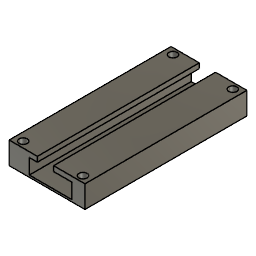
Rail (Autodesk Fusion 360 design; units mm, degrees)
part number: 2025-11-19-14-05-20-306
Autodesk Fusion 360 part; units mm, degrees
sketch "Sketch1" plane through (0, 0, 0) normal (0, 0, 1) x (1, 0, 0)
  line L0 (0, 0) -> (95.25, 0)
  line L1 (95.25, 0) -> (95.25, 203.2)
  line L2 (95.25, 203.2) -> (0, 203.2)
  line L3 (0, 203.2) -> (0, 0)
  dimension "d1" = 95.25
  dimension "d2" = 203.2
  constraint horizontal L0
  constraint vertical L1
  constraint horizontal L2
  constraint vertical L3
  constraint coincident L0.start L3.end
  measures "d1" distance of L0.start L0.end
  measures "d2" distance of L0.start L2.end
extrude "Extrude1" add sketch "Sketch1" along normal blind 27.94
sketch "Sketch3" plane through (0, 0, 0) normal (0, -1, 0) x (1, 0, 0)
  line L0 (0, 0) -> (95.25, 0)
  line L1 (95.25, 0) -> (95.25, 27.94)
  line L2 (95.25, 27.94) -> (0, 27.94)
  line L3 (0, 27.94) -> (0, 0)
  line L4 (95.25, 27.94) -> (49.53, 27.94)
  line L5 (35.56, 27.94) -> (55.88, 27.94)
  line L6 (55.88, 27.94) -> (55.88, 15.24)
  line L7 (55.88, 15.24) -> (35.56, 15.24)
  line L8 (35.56, 15.24) -> (35.56, 27.94)
  line L9 (95.25, 19.05) -> (59.69, 19.05)
  line L10 (0, 21.59) -> (25.4, 21.59)
  line L11 (25.4, 21.59) -> (78.74, 21.59)
  line L12 (78.74, 21.59) -> (78.74, 2.54)
  line L13 (78.74, 2.54) -> (25.4, 2.54)
  line L14 (25.4, 2.54) -> (25.4, 21.59)
  dimension "d21" = 45.72
  dimension "d22" = 12.7
  dimension "d29" = 53.34
  dimension "d30" = 20.32
  dimension "d55" = 19.05
  dimension "d56" = 2.54
  dimension "d57" = 15.24
  dimension "d58" = 35.56
  dimension "d59" = 25.4
  constraint coincident L1.end L2.start
  constraint perpendicular L1 L4
  constraint horizontal L5
  constraint vertical L6
  constraint horizontal L7
  constraint vertical L8
  constraint coincident L1 L9.start
  constraint perpendicular L1 L9
  constraint coincident L3 L10.start
  constraint perpendicular L3 L10
  constraint horizontal L11
  constraint vertical L12
  constraint horizontal L13
  constraint vertical L14
  measures "d21" distance of L1.end L4.end
  measures "d22" distance of L5.start L7.end
  measures "d29" distance of L12.end L13.end
  measures "d30" distance of L5.start L5.end
  measures "d55" distance of L11.end L12.end
  measures "d56" distance of L0 L13
  measures "d57" distance of L0 L7
  measures "d58" distance of L3 L8
  measures "d59" distance of L3 L14
extrude "Extrude3" cut sketch "Sketch3" against normal blind 241.3 contours L6 L7 L8 L11 L12 L13 L14 | L2 L4 L5 L6 L8 L11 | L6 L7 L8 L11
sketch "Sketch5" plane through (0, 0, 27.94) normal (0, 0, 1) x (-1, 0, 0)
  line L0 (-35.56, -203.2) -> (0, -203.2)
  line L1 (0, -203.2) -> (0, 0)
  line L2 (0, 0) -> (-35.56, 0)
  circle A0 centre (-10.16, -7.62) radius 2.54
  circle A1 centre (-10.16, -195.58) radius 2.54
  line L3 (-35.56, 0) -> (-35.56, -203.2)
  dimension "d31" = 5.08
  dimension "d32" = 7.62
  dimension "d33" = 5.08
  dimension "d34" = 10.16
  dimension "d35" = 7.62
  dimension "d41" = 10.16
  measures "d31" diameter of A0
  measures "d32" distance of L2 A0.centre
  measures "d33" diameter of A1
  measures "d34" distance of L1 A1.centre
  measures "d35" distance of L0 A1.centre
  measures "d41" distance of L1 A0.centre
hole "Hole1" at (10.16, 195.58, 27.94) at (10.16, 7.62, 27.94) direction (0, 0, -1) diameter 3.81 depth 48.26 tip angle 118 counterbore diameter 10.16 counterbore depth 19.05
sketch "Sketch6" plane through (0, 0, 27.94) normal (0, 0, 1) x (-1, 0, 0)
  line L0 (-55.88, 0) -> (-95.25, 0)
  line L1 (-95.25, 0) -> (-95.25, -203.2)
  line L2 (-95.25, -203.2) -> (-55.88, -203.2)
  circle A0 centre (-85.09, -7.62) radius 2.54
  circle A1 centre (-85.09, -195.58) radius 2.54
  line L3 (-55.88, -203.2) -> (-55.88, 0)
  dimension "d42" = 5.08
  dimension "d43" = 10.16
  dimension "d44" = 7.62
  dimension "d45" = 5.08
  dimension "d46" = 7.62
  dimension "d47" = 10.16
  measures "d42" diameter of A0
  measures "d43" distance of L1 A0.centre
  measures "d44" distance of L0 A0.centre
  measures "d45" diameter of A1
  measures "d46" distance of L2 A1.centre
  measures "d47" distance of L1 A1.centre
hole "Hole2" at (85.09, 7.62, 27.94) at (85.09, 195.58, 27.94) direction (0, 0, -1) diameter 3.81 depth 45.72 tip angle 118 counterbore diameter 10.16 counterbore depth 19.05
